Autodesk Fusion 360 part; units mm, degrees
(part 3 of 4)
  point P30 (48.244, 24.05)
  point P31 (62.214, 24.05)
  point P32 (118.094, 24.05)
  point P33 (76.184, 24.05)
  point P34 (90.154, 24.05)
  point P35 (104.124, 24.05)
  point P36 (54.673, 10.08)
  point P37 (12.673, 10.08)
  point P38 (26.673, 10.08)
  point P39 (40.673, 10.08)
  point P40 (68.673, 10.08)
  point P41 (82.673, 10.08)
  point P42 (96.673, 10.08)
  point P43 (110.673, 10.08)
  point P44 (124.673, 10.08)
  point P45 (138.673, 10.08)
  point P46 (132.064, 24.05)
  point P47 (146.034, 24.05)
  point P48 (19.024, 24.05)
  point P49 (34.274, 24.05)
  point P50 (48.244, 24.05)
  point P51 (62.214, 24.05)
  point P52 (76.184, 24.05)
  point P53 (90.154, 24.05)
  point P54 (104.124, 24.05)
  point P55 (118.094, 24.05)
  point P56 (146.034, 24.05)
  point P57 (138.673, 10.08)
  point P58 (124.673, 10.08)
  point P59 (110.673, 10.08)
  point P60 (96.673, 10.08)
  point P61 (82.673, 10.08)
  point P62 (68.673, 10.08)
  point P63 (54.673, 10.08)
  point P64 (40.673, 10.08)
  point P65 (26.673, 10.08)
  point P66 (12.673, 10.08)
  point P67 (132.064, 24.05)
  dimension "d105" = 2.7
  dimension "d106" = 2
  dimension "d371" = 1.05
  dimension "d372" = 2.7
  dimension "d373" = 2
  dimension "d374" = 1.05
  dimension "d375" = 2.7
  dimension "d376" = 2
  dimension "d377" = 1.05
  dimension "d378" = 2.7
  dimension "d379" = 2
  dimension "d380" = 1.05
  dimension "d381" = 2.7
  dimension "d382" = 2
  dimension "d383" = 1.05
  dimension "d384" = 2.7
  dimension "d385" = 2
  dimension "d386" = 1.05
  dimension "d387" = 2.7
  dimension "d388" = 2
  dimension "d389" = 1.05
  dimension "d390" = 2.7
  dimension "d391" = 2
  dimension "d392" = 1.05
  dimension "d393" = 2.7
  dimension "d394" = 2
  dimension "d395" = 1.05
  dimension "d396" = 2.7
  dimension "d397" = 2
  dimension "d398" = 1.05
  dimension "d504" = 2.7
  dimension "d505" = 2
  dimension "d506" = 1.05
  dimension "d507" = 2.7
  dimension "d508" = 2
  dimension "d509" = 1.05
  dimension "d510" = 2.7
  dimension "d511" = 2
  dimension "d512" = 1.05
  dimension "d513" = 2.7
  dimension "d514" = 2
  dimension "d515" = 1.05
  dimension "d516" = 2.7
  dimension "d517" = 2
  dimension "d518" = 1.05
  dimension "d519" = 2.7
  dimension "d520" = 2
  dimension "d521" = 1.05
  dimension "d522" = 2.7
  dimension "d523" = 2
  dimension "d524" = 1.05
  dimension "d525" = 2.7
  dimension "d526" = 2
  dimension "d527" = 1.05
  dimension "d528" = 2.7
  dimension "d529" = 2
  dimension "d530" = 1.05
  dimension "d531" = 2.7
  dimension "d532" = 2
  dimension "d533" = 1.05
  dimension "d568" = 2.7
  dimension "d569" = 2
  dimension "d570" = 1.05
  dimension "d571" = 2.7
  dimension "d572" = 2
  dimension "d573" = 1.05
  dimension "d574" = 2.7
  dimension "d575" = 2
  dimension "d576" = 1.05
  dimension "d577" = 2.7
  dimension "d578" = 2
  dimension "d579" = 1.05
  dimension "d580" = 2.7
  dimension "d581" = 2
  dimension "d582" = 1.05
  dimension "d583" = 2.7
  dimension "d584" = 2
  dimension "d585" = 1.05
  dimension "d586" = 2.7
  dimension "d587" = 2
  dimension "d588" = 1.05
  dimension "d589" = 2.7
  dimension "d590" = 2
  dimension "d591" = 1.05
  dimension "d592" = 2.7
  dimension "d593" = 2
  dimension "d594" = 1.05
  dimension "d595" = 2.7
  dimension "d596" = 2
  dimension "d597" = 1.05
  dimension "d598" = 2.7
  dimension "d599" = 2
  dimension "d600" = 1.05
  dimension "d601" = 2.7
  dimension "d602" = 2
  dimension "d603" = 1.05
  dimension "d604" = 2.7
  dimension "d605" = 2
  dimension "d606" = 1.05
  dimension "d607" = 2.7
  dimension "d608" = 2
  dimension "d609" = 1.05
  dimension "d610" = 2.7
  dimension "d611" = 2
  dimension "d612" = 1.05
  dimension "d613" = 2.7
  dimension "d614" = 2
  dimension "d615" = 1.05
  dimension "d616" = 2.7
  dimension "d617" = 2
  dimension "d618" = 1.05
  dimension "d619" = 2.7
  dimension "d620" = 2
  dimension "d621" = 1.05
  dimension "d622" = 2.7
  dimension "d623" = 2
  dimension "d624" = 1.05
  dimension "d625" = 2.7
  dimension "d626" = 2
  dimension "d627" = 1.05
  constraint midpoint L0 L4.start
  constraint midpoint L2 L4.end
  constraint midpoint L1 L5.start
  constraint midpoint L3 L5.end
  constraint vertical L6
  constraint perpendicular L5 L7
  constraint perpendicular L4 L8
  constraint perpendicular L4 L9
  constraint perpendicular L4 L11
  constraint perpendicular L7 L14
  constraint perpendicular L5 L17
  constraint equal L6 L8
  constraint equal L8 L9
  constraint equal L7 L8
  constraint symmetric L4 L8.start L8.end
  constraint symmetric L4 L10.end L11.end
  constraint symmetric L4 L9.start L9.end
  constraint symmetric L4 L13.end L14.end
  constraint symmetric L5 L6.start L6.end
  constraint symmetric L5 L16.end L17.end
  constraint symmetric L5 L7.start L7.end
  constraint collinear L0 L8
  constraint equal L11 L17
  constraint collinear L3 L6
  constraint collinear L2 L9
  constraint collinear L1 L7
  constraint equal L14 L17
  constraint parallel L7 L20
  constraint equal L17 L20
  constraint symmetric L5 L19.end L20.end
  constraint coincident L6 L22.end
  constraint coincident L3 L22.end
  constraint perpendicular L6 L22
  constraint coincident L8 L23.end
  constraint coincident L0 L23.end
  constraint coincident L9 L24.end
  constraint coincident L2 L24.end
  constraint perpendicular L9 L24
  constraint perpendicular L8 L23
  constraint coincident L7 L25.end
  constraint coincident L1 L25.end
  constraint perpendicular L7 L25
  constraint equal L23 L25
  constraint equal L22 L23
  constraint equal L23 L24
  constraint tangent L7 A0
  constraint tangent L6 A0
  constraint tangent L8 A0
  constraint vertical L27
  constraint perpendicular L38 L39
  constraint perpendicular L43 L46
  constraint perpendicular L28 L46
  constraint perpendicular L46 L47
  constraint perpendicular L34 L39
  constraint perpendicular L26 L38
  constraint equal L27 L43
  constraint equal L28 L43
  constraint equal L39 L43
  constraint symmetric L37.start L36.end L46
  constraint symmetric L37.end L32.start L46
  constraint symmetric L28.start L28.end L46
  constraint symmetric L34.start L34.end L46
  constraint symmetric L27.start L27.end L38
  constraint symmetric L26.end L26.start L38
  constraint symmetric L35.start L30.end L38
  constraint equal L26 L47
  constraint equal L26 L34
  constraint parallel L33 L39
  constraint equal L26 L33
  constraint symmetric L33.start L30.start L38
  constraint coincident L29.end L27
  constraint perpendicular L27 L29
  constraint coincident L32.end L43
  constraint coincident L41.end L28
  constraint perpendicular L28 L41
  constraint perpendicular L32 L43
  constraint coincident L42.end L39
  constraint perpendicular L39 L42
  constraint equal L32 L42
  constraint equal L29 L32
  constraint equal L32 L41
  constraint tangent L39 A1
  constraint tangent L27 A1
  constraint tangent L43 A1
  constraint coincident L38.end A1
  constraint coincident L38.start A1
  constraint coincident L46.end A1
  constraint coincident L46.start A1
  constraint tangent L28 A1
  constraint coincident P0 L46
  constraint coincident P0 L38
  constraint equal A0 A1
  constraint vertical L50
  constraint perpendicular L65 L67
  constraint perpendicular L52 L53
  constraint perpendicular L53 L61
  constraint perpendicular L53 L56
  constraint perpendicular L59 L67
  constraint perpendicular L54 L65
  constraint equal L50 L52
  constraint equal L52 L61
  constraint equal L52 L67
  constraint symmetric L51.start L48.end L53
  constraint symmetric L48.start L51.end L53
  constraint symmetric L55.end L60.start L53
  constraint symmetric L59.start L49.start L53
  constraint symmetric L50.end L50.start L65
  constraint symmetric L54.start L54.end L65
  constraint symmetric L67.start L66.end L65
  constraint equal L54 L56
  constraint equal L54 L59
  constraint parallel L67 L68
  constraint equal L54 L68
  constraint symmetric L68.start L64.start L65
  constraint coincident L62.end L50
  constraint perpendicular L50 L62
  constraint coincident L63.end L52
  constraint coincident L49.end L61
  constraint perpendicular L49 L61
  constraint perpendicular L52 L63
  constraint coincident L64.end L67
  constraint perpendicular L64 L67
  constraint equal L63 L64
  constraint equal L62 L63
  constraint equal L49 L63
  constraint tangent L67 A2
  constraint tangent L50 A2
  constraint tangent L52 A2
  constraint coincident L65.end A2
  constraint coincident L65.start A2
  constraint coincident L53.end A2
  constraint coincident L53.start A2
  constraint tangent L61 A2
  constraint coincident P1 L53
  constraint coincident P1 L65
  constraint vertical L72
  constraint perpendicular L87 L89
  constraint perpendicular L74 L75
  constraint perpendicular L75 L83
  constraint perpendicular L75 L78
  constraint perpendicular L81 L89
  constraint perpendicular L76 L87
  constraint equal L72 L74
  constraint equal L74 L83
  constraint equal L74 L89
  constraint symmetric L73.start L70.end L75
  constraint symmetric L70.start L73.end L75
  constraint symmetric L77.end L82.start L75
  constraint symmetric L81.start L71.start L75
  constraint symmetric L72.end L72.start L87
  constraint symmetric L76.start L76.end L87
  constraint symmetric L89.start L88.end L87
  constraint equal L76 L78
  constraint equal L76 L81
  constraint parallel L89 L90
  constraint equal L76 L90
  constraint symmetric L90.start L86.start L87
  constraint coincident L84.end L72
  constraint perpendicular L72 L84
  constraint coincident L85.end L74
  constraint coincident L71.end L83
  constraint perpendicular L71 L83
  constraint perpendicular L74 L85
  constraint coincident L86.end L89
  constraint perpendicular L86 L89
  constraint equal L85 L86
  constraint equal L84 L85
  constraint equal L71 L85
  constraint tangent L89 A3
  constraint tangent L72 A3
  constraint tangent L74 A3
  constraint coincident L87.end A3
  constraint coincident L87.start A3
  constraint coincident L75.end A3
  constraint coincident L75.start A3
  constraint tangent L83 A3
  constraint coincident P2 L75
  constraint coincident P2 L87
  constraint vertical L94
  constraint perpendicular L109 L111
  constraint perpendicular L96 L97
  constraint perpendicular L97 L105
  constraint perpendicular L97 L100
  constraint perpendicular L103 L111
  constraint perpendicular L98 L109
  constraint equal L94 L96
  constraint equal L96 L105
  constraint equal L96 L111
  constraint symmetric L95.start L92.end L97
  constraint symmetric L92.start L95.end L97
  constraint symmetric L99.end L104.start L97
  constraint symmetric L103.start L93.start L97
  constraint symmetric L94.end L94.start L109
  constraint symmetric L98.start L98.end L109
  constraint symmetric L111.start L110.end L109
  constraint equal L98 L100
  constraint equal L98 L103
  constraint parallel L111 L112
  constraint equal L98 L112
  constraint symmetric L112.start L108.start L109
  constraint coincident L106.end L94
  constraint perpendicular L94 L106
  constraint coincident L107.end L96
  constraint coincident L93.end L105
  constraint perpendicular L93 L105
  constraint perpendicular L96 L107
  constraint coincident L108.end L111
  constraint perpendicular L108 L111
  constraint equal L107 L108
  constraint equal L106 L107
  constraint equal L93 L107
  constraint tangent L111 A4
  constraint tangent L94 A4
  constraint tangent L96 A4
  constraint coincident L109.end A4
  constraint coincident L109.start A4
  constraint coincident L97.end A4
  constraint coincident L97.start A4
  constraint tangent L105 A4
  constraint coincident P3 L97
  constraint coincident P3 L109
  constraint vertical L116
  constraint perpendicular L131 L133
  constraint perpendicular L118 L119
  constraint perpendicular L119 L127
  constraint perpendicular L119 L122
  constraint perpendicular L125 L133
  constraint perpendicular L120 L131
  constraint equal L116 L118
  constraint equal L118 L127
  constraint equal L118 L133
  constraint symmetric L117.start L114.end L119
  constraint symmetric L114.start L117.end L119
  constraint symmetric L121.end L126.start L119
  constraint symmetric L125.start L115.start L119
  constraint symmetric L116.end L116.start L131
  constraint symmetric L120.start L120.end L131
  constraint symmetric L133.start L132.end L131
  constraint equal L120 L122
  constraint equal L120 L125
  constraint parallel L133 L134
  constraint equal L120 L134
  constraint symmetric L134.start L130.start L131
  constraint coincident L128.end L116
  constraint perpendicular L116 L128
  constraint coincident L129.end L118
  constraint coincident L115.end L127
  constraint perpendicular L115 L127
  constraint perpendicular L118 L129
  constraint coincident L130.end L133
  constraint perpendicular L130 L133
  constraint equal L129 L130
  constraint equal L128 L129
  constraint equal L115 L129
  constraint tangent L133 A5
  constraint tangent L116 A5
  constraint tangent L118 A5
  constraint coincident L131.end A5
  constraint coincident L131.start A5
  constraint coincident L119.end A5
  constraint coincident L119.start A5
  constraint tangent L127 A5
  constraint coincident P4 L119
  constraint coincident P4 L131
  constraint vertical L138
  constraint perpendicular L153 L155
  constraint perpendicular L140 L141
  constraint perpendicular L141 L149
  constraint perpendicular L141 L144
  constraint perpendicular L147 L155
  constraint perpendicular L142 L153
  constraint equal L138 L140
  constraint equal L140 L149
  constraint equal L140 L155
  constraint symmetric L139.start L136.end L141
  constraint symmetric L136.start L139.end L141
  constraint symmetric L143.end L148.start L141
  constraint symmetric L147.start L137.start L141
  constraint symmetric L138.end L138.start L153
  constraint symmetric L142.start L142.end L153
  constraint symmetric L155.start L154.end L153
  constraint equal L142 L144
  constraint equal L142 L147
  constraint parallel L155 L156
  constraint equal L142 L156
  constraint symmetric L156.start L152.start L153
  constraint coincident L150.end L138
  constraint perpendicular L138 L150
  constraint coincident L151.end L140
  constraint coincident L137.end L149
  constraint perpendicular L137 L149
  constraint perpendicular L140 L151
  constraint coincident L152.end L155
  constraint perpendicular L152 L155
  constraint equal L151 L152
  constraint equal L150 L151
  constraint equal L137 L151
  constraint tangent L155 A6
  constraint tangent L138 A6
  constraint tangent L140 A6
  constraint coincident L153.end A6
  constraint coincident L153.start A6
  constraint coincident L141.end A6
  constraint coincident L141.start A6
  constraint tangent L149 A6
  constraint coincident P5 L141
  constraint coincident P5 L153
  constraint vertical L160
  constraint perpendicular L175 L177
  constraint perpendicular L162 L163
  constraint perpendicular L163 L171
  constraint perpendicular L163 L166
  constraint perpendicular L169 L177
  constraint perpendicular L164 L175
  constraint equal L160 L162
  constraint equal L162 L171
  constraint equal L162 L177
  constraint symmetric L161.start L158.end L163
  constraint symmetric L158.start L161.end L163
  constraint symmetric L165.end L170.start L163
  constraint symmetric L169.start L159.start L163
  constraint symmetric L160.end L160.start L175
  constraint symmetric L164.start L164.end L175
  constraint symmetric L177.start L176.end L175
  constraint equal L164 L166
  constraint equal L164 L169
  constraint parallel L177 L178
  constraint equal L164 L178
  constraint symmetric L178.start L174.start L175
  constraint coincident L172.end L160
  constraint perpendicular L160 L172
  constraint coincident L173.end L162
  constraint coincident L159.end L171
  constraint perpendicular L159 L171
  constraint perpendicular L162 L173
  constraint coincident L174.end L177
  constraint perpendicular L174 L177
  constraint equal L173 L174
  constraint equal L172 L173
  constraint equal L159 L173
  constraint tangent L177 A7
  constraint tangent L160 A7
  constraint tangent L162 A7
  constraint coincident L175.end A7
  constraint coincident L175.start A7
  constraint coincident L163.end A7
  constraint coincident L163.start A7
  constraint tangent L171 A7
  constraint coincident P6 L163
  constraint coincident P6 L175
  constraint vertical L182
  constraint perpendicular L197 L199
  constraint perpendicular L184 L185
  constraint perpendicular L185 L193
  constraint perpendicular L185 L188
  constraint perpendicular L191 L199
  constraint perpendicular L186 L197
  constraint equal L182 L184
  constraint equal L184 L193
  constraint equal L184 L199
  constraint symmetric L183.start L180.end L185
  constraint symmetric L180.start L183.end L185
  constraint symmetric L187.end L192.start L185
  constraint symmetric L191.start L181.start L185
  constraint symmetric L182.end L182.start L197
  constraint symmetric L186.start L186.end L197
  constraint symmetric L199.start L198.end L197
  constraint equal L186 L188
  constraint equal L186 L191
  constraint parallel L199 L200
  constraint equal L186 L200
  constraint symmetric L200.start L196.start L197
  constraint coincident L194.end L182
  constraint perpendicular L182 L194
  constraint coincident L195.end L184
  constraint coincident L181.end L193
  constraint perpendicular L181 L193
  constraint perpendicular L184 L195
  constraint coincident L196.end L199
  constraint perpendicular L196 L199
  constraint equal L195 L196
  constraint equal L194 L195
  constraint equal L181 L195
  constraint tangent L199 A8
  constraint tangent L182 A8
  constraint tangent L184 A8
  constraint coincident L197.end A8
  constraint coincident L197.start A8
  constraint coincident L185.end A8
  constraint coincident L185.start A8
  constraint tangent L193 A8
  constraint coincident P7 L185
  constraint coincident P7 L197
  constraint vertical L204
  constraint perpendicular L219 L221
  constraint perpendicular L206 L207
  constraint perpendicular L207 L215
  constraint perpendicular L207 L210
  constraint perpendicular L213 L221
  constraint perpendicular L208 L219
  constraint equal L204 L206
  constraint equal L206 L215
  constraint equal L206 L221
  constraint symmetric L205.start L202.end L207
  constraint symmetric L202.start L205.end L207
  constraint symmetric L209.end L214.start L207
  constraint symmetric L213.start L203.start L207
  constraint symmetric L204.end L204.start L219
  constraint symmetric L208.start L208.end L219
  constraint symmetric L221.start L220.end L219
  constraint equal L208 L210
  constraint equal L208 L213
  constraint parallel L221 L222
  constraint equal L208 L222
  constraint symmetric L222.start L218.start L219
  constraint coincident L216.end L204
  constraint perpendicular L204 L216
  constraint coincident L217.end L206
  constraint coincident L203.end L215
  constraint perpendicular L203 L215
  constraint perpendicular L206 L217
  constraint coincident L218.end L221
  constraint perpendicular L218 L221
  constraint equal L217 L218
  constraint equal L216 L217
  constraint equal L203 L217
  constraint tangent L221 A9
  constraint tangent L204 A9
  constraint tangent L206 A9
  constraint coincident L219.end A9
  constraint coincident L219.start A9
  constraint coincident L207.end A9
  constraint coincident L207.start A9
  constraint tangent L215 A9
  constraint coincident P8 L207
  constraint coincident P8 L219
  constraint coincident P0 A1.centre
  constraint coincident P1 A2.centre
  constraint equal A0 A2
  constraint coincident P2 A3.centre
  constraint equal A0 A3
  constraint coincident P3 A4.centre
  constraint coincident P4 A5.centre
  constraint coincident P5 A6.centre
  constraint coincident P6 A7.centre
  constraint coincident P7 A8.centre
  constraint coincident P8 A9.centre
  constraint equal A0 A4
  constraint equal A0 A9
  constraint equal A0 A8
  constraint equal A0 A7
  constraint equal A0 A6
  constraint equal A0 A5
  constraint vertical L227
  constraint perpendicular L234 L236
  constraint perpendicular L235 L238
  constraint perpendicular L238 L241
  constraint perpendicular L238 L243
  constraint perpendicular L228 L234
  constraint perpendicular L229 L236
  constraint equal L227 L235
  constraint equal L235 L241
  constraint equal L234 L235
  constraint symmetric L224.start L235.end L238
  constraint symmetric L230.start L224.end L238
  constraint symmetric L232.start L237.end L238
  constraint symmetric L228.start L228.end L238
  constraint symmetric L227.end L227.start L236
  constraint symmetric L229.start L229.end L236
  constraint symmetric L234.start L234.end L236
  constraint equal L229 L243
  constraint equal L228 L229
  constraint parallel L226 L234
  constraint equal L226 L229
  constraint symmetric L226.start L225.start L236
  constraint coincident L245.end L227
  constraint perpendicular L227 L245
  constraint coincident L230.end L235
  constraint coincident L233.end L241
  constraint perpendicular L233 L241
  constraint perpendicular L230 L235
  constraint coincident L225.end L234
  constraint perpendicular L225 L234
  constraint equal L225 L230
  constraint equal L230 L245
  constraint equal L230 L233
  constraint tangent A10 L234
  constraint tangent A10 L227
  constraint tangent A10 L235
  constraint coincident L236.end A10
  constraint coincident L236.start A10
  constraint coincident L238.end A10
  constraint coincident L238.start A10
  constraint tangent A10 L241
  constraint coincident P19 L238
  constraint coincident P19 L236
  constraint coincident P19 P9
  constraint vertical L249
  constraint perpendicular L256 L258
  constraint perpendicular L257 L260
  constraint perpendicular L260 L263
  constraint perpendicular L260 L265
  constraint perpendicular L250 L256
  constraint perpendicular L251 L258
  constraint equal L249 L257
  constraint equal L257 L263
  constraint equal L256 L257
  constraint symmetric L246.start L257.end L260
  constraint symmetric L252.start L246.end L260
  constraint symmetric L254.start L259.end L260
  constraint symmetric L250.start L250.end L260
  constraint symmetric L249.end L249.start L258
  constraint symmetric L251.start L251.end L258
  constraint symmetric L256.start L256.end L258
  constraint equal L251 L265
  constraint equal L250 L251
  constraint parallel L248 L256
  constraint equal L248 L251
  constraint symmetric L248.start L247.start L258
  constraint coincident L267.end L249
  constraint perpendicular L249 L267
  constraint coincident L252.end L257
  constraint coincident L255.end L263
  constraint perpendicular L255 L263
  constraint perpendicular L252 L257
  constraint coincident L247.end L256
  constraint perpendicular L247 L256
  constraint equal L247 L252
  constraint equal L252 L267
  constraint equal L252 L255
  constraint tangent A11 L256
  constraint tangent A11 L249
  constraint tangent A11 L257
  constraint coincident L258.end A11
  constraint coincident L258.start A11
  constraint coincident L260.end A11
  constraint coincident L260.start A11
  constraint tangent A11 L263
  constraint coincident P27 L260
  constraint coincident P27 L258
  constraint coincident P27 P10
  constraint vertical L271
  constraint perpendicular L278 L280
  constraint perpendicular L279 L282
  constraint perpendicular L282 L285
  constraint perpendicular L282 L287
  constraint perpendicular L272 L278
  constraint perpendicular L273 L280
  constraint equal L271 L279
  constraint equal L279 L285
  constraint equal L278 L279
  constraint symmetric L268.start L279.end L282
  constraint symmetric L274.start L268.end L282
  constraint symmetric L276.start L281.end L282
  constraint symmetric L272.start L272.end L282
  constraint symmetric L271.end L271.start L280
  constraint symmetric L273.start L273.end L280
  constraint symmetric L278.start L278.end L280
  constraint equal L273 L287
  constraint equal L272 L273
  constraint parallel L270 L278
  constraint equal L270 L273
  constraint symmetric L270.start L269.start L280
  constraint coincident L289.end L271
  constraint perpendicular L271 L289
  constraint coincident L274.end L279
  constraint coincident L277.end L285
  constraint perpendicular L277 L285
  constraint perpendicular L274 L279
  constraint coincident L269.end L278
  constraint perpendicular L269 L278
  constraint equal L269 L274
  constraint equal L274 L289
  constraint equal L274 L277
  constraint tangent A12 L278
  constraint tangent A12 L271
  constraint tangent A12 L279
  constraint coincident L280.end A12
  constraint coincident L280.start A12
  constraint coincident L282.end A12
  constraint coincident L282.start A12
  constraint tangent A12 L285
  constraint coincident P26 L282
  constraint coincident P26 L280
  constraint coincident P26 P11
  constraint vertical L293
  constraint perpendicular L300 L302
  constraint perpendicular L301 L304
  constraint perpendicular L304 L307
  constraint perpendicular L304 L309
  constraint perpendicular L294 L300
  constraint perpendicular L295 L302
  constraint equal L293 L301
  constraint equal L301 L307
  constraint equal L300 L301
  constraint symmetric L290.start L301.end L304
  constraint symmetric L296.start L290.end L304
  constraint symmetric L298.start L303.end L304
  constraint symmetric L294.start L294.end L304
  constraint symmetric L293.end L293.start L302
  constraint symmetric L295.start L295.end L302
  constraint symmetric L300.start L300.end L302
  constraint equal L295 L309
  constraint equal L294 L295
  constraint parallel L292 L300
  constraint equal L292 L295
  constraint symmetric L292.start L291.start L302
  constraint coincident L311.end L293
  constraint perpendicular L293 L311
  constraint coincident L296.end L301
  constraint coincident L299.end L307
  constraint perpendicular L299 L307
  constraint perpendicular L296 L301
  constraint coincident L291.end L300
  constraint perpendicular L291 L300
  constraint equal L291 L296
  constraint equal L296 L311
  constraint equal L296 L299
  constraint tangent A13 L300
  constraint tangent A13 L293
  constraint tangent A13 L301
  constraint coincident L302.end A13
  constraint coincident L302.start A13
  constraint coincident L304.end A13
  constraint coincident L304.start A13
  constraint tangent A13 L307
  constraint coincident P25 L304
  constraint coincident P25 L302
  constraint coincident P25 P12
  constraint vertical L315
  constraint perpendicular L322 L324
  constraint perpendicular L323 L326
  constraint perpendicular L326 L329
  constraint perpendicular L326 L331
  constraint perpendicular L316 L322
  constraint perpendicular L317 L324
  constraint equal L315 L323
  constraint equal L323 L329
  constraint equal L322 L323
  constraint symmetric L312.start L323.end L326
  constraint symmetric L318.start L312.end L326
  constraint symmetric L320.start L325.end L326
  constraint symmetric L316.start L316.end L326
  constraint symmetric L315.end L315.start L324
  constraint symmetric L317.start L317.end L324
  constraint symmetric L322.start L322.end L324
  constraint equal L317 L331
  constraint equal L316 L317
  constraint parallel L314 L322
  constraint equal L314 L317
  constraint symmetric L314.start L313.start L324
  constraint coincident L333.end L315
  constraint perpendicular L315 L333
  constraint coincident L318.end L323
  constraint coincident L321.end L329
  constraint perpendicular L321 L329
  constraint perpendicular L318 L323
  constraint coincident L313.end L322
  constraint perpendicular L313 L322
  constraint equal L313 L318
  constraint equal L318 L333
  constraint equal L318 L321
  constraint tangent A14 L322
  constraint tangent A14 L315
  constraint tangent A14 L323
  constraint coincident L324.end A14
  constraint coincident L324.start A14
  constraint coincident L326.end A14
  constraint coincident L326.start A14
  constraint tangent A14 L329
  constraint coincident P18 L326
  constraint coincident P18 L324
  constraint vertical L337
  constraint perpendicular L344 L346
  constraint perpendicular L345 L348
  constraint perpendicular L348 L351
  constraint perpendicular L348 L353
  constraint perpendicular L338 L344
  constraint perpendicular L339 L346
  constraint equal L337 L345
  constraint equal L345 L351
  constraint equal L344 L345
  constraint symmetric L334.start L345.end L348
  constraint symmetric L340.start L334.end L348
  constraint symmetric L342.start L347.end L348
  constraint symmetric L338.start L338.end L348
  constraint symmetric L337.end L337.start L346
  constraint symmetric L339.start L339.end L346
  constraint symmetric L344.start L344.end L346
  constraint equal L339 L353
  constraint equal L338 L339
  constraint parallel L336 L344
  constraint equal L336 L339
  constraint symmetric L336.start L335.start L346
  constraint coincident L355.end L337
  constraint perpendicular L337 L355
  constraint coincident L340.end L345
  constraint coincident L343.end L351
  constraint perpendicular L343 L351
  constraint perpendicular L340 L345
  constraint coincident L335.end L344
  constraint perpendicular L335 L344
  constraint equal L335 L340
  constraint equal L340 L355
  constraint equal L340 L343
  constraint tangent A15 L344
  constraint tangent A15 L337
  constraint tangent A15 L345
  constraint coincident L346.end A15
  constraint coincident L346.start A15
  constraint coincident L348.end A15
  constraint coincident L348.start A15
  constraint tangent A15 L351
  constraint coincident P24 L348
  constraint coincident P24 L346
  constraint coincident P24 P13
  constraint vertical L359
  constraint perpendicular L366 L368
  constraint perpendicular L367 L370
  constraint perpendicular L370 L373
  constraint perpendicular L370 L375
  constraint perpendicular L360 L366
  constraint perpendicular L361 L368
  constraint equal L359 L367
  constraint equal L367 L373
  constraint equal L366 L367
  constraint symmetric L356.start L367.end L370
  constraint symmetric L362.start L356.end L370
  constraint symmetric L364.start L369.end L370
  constraint symmetric L360.start L360.end L370
  constraint symmetric L359.end L359.start L368
  constraint symmetric L361.start L361.end L368
  constraint symmetric L366.start L366.end L368
  constraint equal L361 L375
  constraint equal L360 L361
  constraint parallel L358 L366
  constraint equal L358 L361
  constraint symmetric L358.start L357.start L368
  constraint coincident L377.end L359
  constraint perpendicular L359 L377
  constraint coincident L362.end L367
  constraint coincident L365.end L373
  constraint perpendicular L365 L373
  constraint perpendicular L362 L367
  constraint coincident L357.end L366
  constraint perpendicular L357 L366
  constraint equal L357 L362
  constraint equal L362 L377
  constraint equal L362 L365
  constraint tangent A16 L366
  constraint tangent A16 L359
  constraint tangent A16 L367
  constraint coincident L368.end A16
  constraint coincident L368.start A16
  constraint coincident L370.end A16
  constraint coincident L370.start A16
  constraint tangent A16 L373
  constraint coincident P23 L370
  constraint coincident P23 L368
  constraint coincident P23 P14
  constraint vertical L381
  constraint perpendicular L388 L390
  constraint perpendicular L389 L392
  constraint perpendicular L392 L395
  constraint perpendicular L392 L397
  constraint perpendicular L382 L388
  constraint perpendicular L383 L390
  constraint equal L381 L389
  constraint equal L389 L395
  constraint equal L388 L389
  constraint symmetric L378.start L389.end L392
  constraint symmetric L384.start L378.end L392
  constraint symmetric L386.start L391.end L392
  constraint symmetric L382.start L382.end L392
  constraint symmetric L381.end L381.start L390
  constraint symmetric L383.start L383.end L390
  constraint symmetric L388.start L388.end L390
  constraint equal L383 L397
  constraint equal L382 L383
  constraint parallel L380 L388
  constraint equal L380 L383
  constraint symmetric L380.start L379.start L390
  constraint coincident L399.end L381
  constraint perpendicular L381 L399
  constraint coincident L384.end L389
  constraint coincident L387.end L395
  constraint perpendicular L387 L395
  constraint perpendicular L384 L389
  constraint coincident L379.end L388
  constraint perpendicular L379 L388
  constraint equal L379 L384
  constraint equal L384 L399
  constraint equal L384 L387
  constraint tangent A17 L388
  constraint tangent A17 L381
  constraint tangent A17 L389
  constraint coincident L390.end A17
  constraint coincident L390.start A17
  constraint coincident L392.end A17
  constraint coincident L392.start A17
  constraint tangent A17 L395
  constraint coincident P22 L392
  constraint coincident P22 L390
  constraint coincident P22 P15
  constraint vertical L403
  constraint perpendicular L410 L412
  constraint perpendicular L411 L414
  constraint perpendicular L414 L417
  constraint perpendicular L414 L419
  constraint perpendicular L404 L410
  constraint perpendicular L405 L412
  constraint equal L403 L411
  constraint equal L411 L417
  constraint equal L410 L411
  constraint symmetric L400.start L411.end L414
  constraint symmetric L406.start L400.end L414
  constraint symmetric L408.start L413.end L414
  constraint symmetric L404.start L404.end L414
  constraint symmetric L403.end L403.start L412
  constraint symmetric L405.start L405.end L412
  constraint symmetric L410.start L410.end L412
  constraint equal L405 L419
  constraint equal L404 L405
  constraint parallel L402 L410
  constraint equal L402 L405
  constraint symmetric L402.start L401.start L412
  constraint coincident L421.end L403
  constraint perpendicular L403 L421
  constraint coincident L406.end L411
  constraint coincident L409.end L417
  constraint perpendicular L409 L417
  constraint perpendicular L406 L411
  constraint coincident L401.end L410
  constraint perpendicular L401 L410
  constraint equal L401 L406
  constraint equal L406 L421
  constraint equal L406 L409
  constraint tangent A18 L410
  constraint tangent A18 L403
  constraint tangent A18 L411
  constraint coincident L412.end A18
  constraint coincident L412.start A18
  constraint coincident L414.end A18
  constraint coincident L414.start A18
  constraint tangent A18 L417
  constraint coincident P21 L414
  constraint coincident P21 L412
  constraint coincident P21 P16
  constraint vertical L425
  constraint perpendicular L432 L434
  constraint perpendicular L433 L436
  constraint perpendicular L436 L439
  constraint perpendicular L436 L441
  constraint perpendicular L426 L432
  constraint perpendicular L427 L434
  constraint equal L425 L433
  constraint equal L433 L439
  constraint equal L432 L433
  constraint symmetric L422.start L433.end L436
  constraint symmetric L428.start L422.end L436
  constraint symmetric L430.start L435.end L436
  constraint symmetric L426.start L426.end L436
  constraint symmetric L425.end L425.start L434
  constraint symmetric L427.start L427.end L434
  constraint symmetric L432.start L432.end L434
  constraint equal L427 L441
  constraint equal L426 L427
  constraint parallel L424 L432
  constraint equal L424 L427
  constraint symmetric L424.start L423.start L434
  constraint coincident L443.end L425
  constraint perpendicular L425 L443
  constraint coincident L428.end L433
  constraint coincident L431.end L439
  constraint perpendicular L431 L439
  constraint perpendicular L428 L433
  constraint coincident L423.end L432
  constraint perpendicular L423 L432
  constraint equal L423 L428
  constraint equal L428 L443
  constraint equal L428 L431
  constraint tangent A19 L432
  constraint tangent A19 L425
  constraint tangent A19 L433
  constraint coincident L434.end A19
  constraint coincident L434.start A19
  constraint coincident L436.end A19
  constraint coincident L436.start A19
  constraint tangent A19 L439
  constraint coincident P20 L436
  constraint coincident P20 L434
  constraint coincident P20 P17
  constraint coincident P18 A14.centre
  constraint equal A14 A20
  constraint equal A10 A21
  constraint equal A11 A22
  constraint equal A12 A23
  constraint equal A13 A24
  constraint equal A15 A25
  constraint equal A16 A26
  constraint equal A17 A27
  constraint equal A18 A28
  constraint equal A19 A29
  constraint vertical L464
  constraint perpendicular L446 L448
  constraint perpendicular L452 L463
  constraint perpendicular L453 L463
  constraint perpendicular L462 L463
  constraint perpendicular L448 L456
  constraint perpendicular L446 L465
  constraint equal L452 L464
  constraint equal L452 L453
  constraint equal L448 L452
  constraint symmetric L450.end L452.start L463
  constraint symmetric L450.start L459.end L463
  constraint symmetric L447.start L444.end L463
  constraint symmetric L444.start L447.end L463
  constraint symmetric L460.end L461.start L446
  constraint symmetric L461.end L458.start L446
  constraint symmetric L448.start L448.end L446
  constraint equal L462 L465
  constraint equal L456 L465
  constraint parallel L448 L451
  constraint equal L451 L465
  constraint symmetric L451.end L449.end L446
  constraint coincident L458.end L464
  constraint perpendicular L458 L464
  constraint coincident L457.end L452
  constraint coincident L445.end L453
  constraint perpendicular L445 L453
  constraint perpendicular L452 L457
  constraint coincident L454.end L448
  constraint perpendicular L448 L454
  constraint equal L454 L457
  constraint equal L457 L458
  constraint equal L445 L457
  constraint tangent L448 A30
  constraint tangent A30 L464
  constraint tangent L452 A30
  constraint coincident L446.end A30
  constraint coincident L446.start A30
  constraint coincident L463.end A30
  constraint coincident L463.start A30
  constraint tangent A30 L453
  constraint coincident P48 L463
  constraint coincident P48 L446
  constraint coincident P48 P28
  constraint vertical L474
  constraint perpendicular L468 L472
  constraint perpendicular L481 L485
  constraint perpendicular L470 L485
  constraint perpendicular L482 L485
  constraint perpendicular L472 L480
  constraint perpendicular L468 L475
  constraint equal L474 L481
  constraint equal L470 L481
  constraint equal L472 L481
  constraint symmetric L477.end L481.start L485
  constraint symmetric L477.start L482.start L485
  constraint symmetric L470.end L466.end L485
  constraint symmetric L466.start L476.end L485
  constraint symmetric L474.start L469.start L468
  constraint symmetric L469.end L475.end L468
  constraint symmetric L472.start L471.end L468
  constraint equal L475 L482
  constraint equal L475 L480
  constraint parallel L472 L487
  constraint equal L475 L487
  constraint symmetric L467.start L473.end L468
  constraint coincident L479.end L474
  constraint perpendicular L474 L479
  constraint coincident L478.end L481
  constraint coincident L483.end L470
  constraint perpendicular L470 L483
  constraint perpendicular L478 L481
  constraint coincident L467.end L472
  constraint perpendicular L467 L472
  constraint equal L467 L478
  constraint equal L478 L479
  constraint equal L478 L483
  constraint tangent L472 A31
  constraint tangent L474 A31
  constraint tangent A31 L481
  constraint coincident L468.end A31
  constraint coincident L468.start A31
  constraint coincident L485.end A31
  constraint coincident L485.start A31
  constraint tangent L470 A31
  constraint coincident P49 L485
  constraint coincident P49 L468
  constraint coincident P49 P29
  constraint vertical L522
  constraint perpendicular L488 L530
  constraint perpendicular L499 L526
  constraint perpendicular L492 L526
  constraint perpendicular L510 L526
  constraint perpendicular L488 L503
  constraint perpendicular L505 L530
  constraint equal L499 L522
  constraint equal L492 L499
  constraint equal L488 L499
  constraint symmetric L495.end L499.start L526
  constraint symmetric L495.start L510.start L526
  constraint symmetric L492.end L492.start L526
  constraint symmetric L503.end L497.end L526
  constraint symmetric L506.end L508.start L530
  constraint symmetric L505.start L504.start L530
  constraint symmetric L488.start L488.end L530
  constraint equal L505 L510
  constraint equal L503 L505
  constraint parallel L488 L493
  constraint equal L493 L505
  constraint symmetric L493.end L491.end L530
  constraint coincident L504.end L522
  constraint perpendicular L504 L522
  constraint coincident L528.end L499
  constraint coincident L519.end L492
  constraint perpendicular L492 L519
  constraint perpendicular L499 L528
  constraint coincident L498.end L488
  constraint perpendicular L488 L498
  constraint equal L498 L528
  constraint equal L504 L528
  constraint equal L519 L528
  constraint tangent L488 A32
  constraint tangent A32 L522
  constraint tangent L499 A32
  constraint coincident L530.end A32
  constraint coincident L530.start A32
  constraint coincident L526.end A32
  constraint coincident L526.start A32
  constraint tangent L492 A32
  constraint coincident P50 L526
  constraint coincident P50 L530
  constraint coincident P50 P30
  constraint vertical L517
  constraint perpendicular L489 L524
  constraint perpendicular L513 L520
  constraint perpendicular L501 L520
  constraint perpendicular L496 L520
  constraint perpendicular L507 L524
  constraint perpendicular L489 L502
  constraint equal L513 L517
  constraint equal L501 L513
  constraint equal L513 L524
  constraint symmetric L513.start L513.end L520
  constraint symmetric L496.start L496.end L520
  constraint symmetric L494.end L501.end L520
  constraint symmetric L494.start L507.start L520
  constraint symmetric L500.end L509.start L489
  constraint symmetric L502.start L490.start L489
  constraint symmetric L511.end L516.start L489
  constraint equal L496 L502
  constraint equal L502 L507
  constraint parallel L524 L525
  constraint equal L502 L525
  constraint symmetric L511.start L516.end L489
  constraint coincident L490.end L517
  constraint perpendicular L490 L517
  constraint coincident L523.end L513
  constraint coincident L521.end L501
  constraint perpendicular L501 L521
  constraint perpendicular L513 L523
  constraint coincident L514.end L524
  constraint perpendicular L514 L524
  constraint equal L514 L523
  constraint equal L490 L523
  constraint equal L521 L523
  constraint tangent A33 L524
  constraint tangent L517 A33
  constraint tangent L513 A33
  constraint coincident L489.end A33
  constraint coincident L489.start A33
  constraint coincident L520.end A33
  constraint coincident L520.start A33
  constraint tangent L501 A33
  constraint coincident P51 L520
  constraint coincident P51 L489
  constraint coincident P51 P31
  constraint vertical L574
  constraint perpendicular L535 L578
  constraint perpendicular L559 L581
  constraint perpendicular L554 L559
  constraint perpendicular L559 L588
  constraint perpendicular L535 L594
  constraint perpendicular L578 L598
  constraint equal L574 L581
  constraint equal L554 L581
  constraint equal L535 L581
  constraint symmetric L542.end L581.start L559
  constraint symmetric L542.start L588.start L559
  constraint symmetric L548.start L554.start L559
  constraint symmetric L582.start L548.end L559
  constraint symmetric L569.end L574.end L578
  constraint symmetric L575.end L569.start L578
  constraint symmetric L535.start L533.end L578
  constraint equal L588 L598
  constraint equal L594 L598
  constraint parallel L535 L560
  constraint equal L560 L598
  constraint symmetric L533.start L545.end L578
  constraint coincident L583.end L574
  constraint perpendicular L574 L583
  constraint coincident L561.end L581
  constraint coincident L582.end L554
  constraint perpendicular L554 L582
  constraint perpendicular L561 L581
  constraint coincident L534.end L535
  constraint perpendicular L534 L535
  constraint equal L534 L561
  constraint equal L561 L583
  constraint equal L561 L582
  constraint tangent L535 A36
  constraint tangent L574 A36
  constraint tangent L581 A36
  constraint coincident L578.end A36
  constraint coincident L578.start A36
  constraint coincident L559.end A36
  constraint coincident L559.start A36
  constraint tangent L554 A36
  constraint coincident P52 L559
  constraint coincident P52 L578
  constraint coincident P52 P33
  constraint vertical L602
  constraint perpendicular L532 L536
  constraint perpendicular L553 L576
  constraint perpendicular L553 L571
  constraint perpendicular L553 L609
  constraint perpendicular L532 L566
  constraint perpendicular L536 L567
  constraint equal L576 L602
  constraint equal L571 L576
  constraint equal L532 L576
  constraint symmetric L576.start L539.end L553
  constraint symmetric L601.end L539.start L553
  constraint symmetric L547.end L550.start L553
  constraint symmetric L547.start L550.end L553
  constraint symmetric L538.end L556.start L536
  constraint symmetric L556.end L538.start L536
  constraint symmetric L532.end L532.start L536
  constraint equal L567 L609
  constraint equal L566 L567
  constraint parallel L532 L570
  constraint equal L567 L570
  constraint symmetric L570.end L570.start L536
  constraint coincident L558.end L602
  constraint perpendicular L558 L602
  constraint coincident L540.end L576
  constraint coincident L551.end L571
  constraint perpendicular L551 L571
  constraint perpendicular L540 L576
  constraint coincident L573.end L532
  constraint perpendicular L532 L573
  constraint equal L540 L573
  constraint equal L540 L558
  constraint equal L540 L551
  constraint tangent L532 A35
  constraint tangent A35 L602
  constraint tangent A35 L576
  constraint coincident L536.end A35
  constraint coincident L536.start A35
  constraint coincident L553.end A35
  constraint coincident L553.start A35
  constraint tangent A35 L571
  constraint coincident P53 L553
  constraint coincident P53 L536
  constraint coincident P53 P34
  constraint vertical L564
  constraint perpendicular L546 L600
  constraint perpendicular L549 L580
  constraint perpendicular L580 L590
  constraint perpendicular L562 L580
  constraint perpendicular L544 L546
  constraint perpendicular L579 L600
  constraint equal L549 L564
  constraint equal L549 L590
  constraint equal L546 L549
  constraint symmetric L549.end L549.start L580
  constraint symmetric L555.start L562.start L580
  constraint symmetric L537.start L563.end L580
  constraint symmetric L544.end L537.end L580
  constraint symmetric L541.end L543.start L600
  constraint symmetric L543.end L541.start L600
  constraint symmetric L546.end L546.start L600
  constraint equal L562 L579
  constraint equal L544 L579
  constraint parallel L546 L585
  constraint equal L579 L585
  constraint symmetric L552.start L568.end L600
  constraint coincident L557.end L564
  constraint perpendicular L557 L564
  constraint coincident L555.end L549
  constraint coincident L599.end L590
  constraint perpendicular L590 L599
  constraint perpendicular L549 L555
  constraint coincident L552.end L546
  constraint perpendicular L546 L552
  constraint equal L552 L555
  constraint equal L555 L557
  constraint equal L555 L599
  constraint tangent A34 L546
  constraint tangent A34 L564
  constraint tangent A34 L549
  constraint coincident L600.end A34
  constraint coincident L600.start A34
  constraint coincident L580.end A34
  constraint coincident L580.start A34
  constraint tangent A34 L590
  constraint coincident P54 L580
  constraint coincident P54 L600
  constraint coincident P54 P35
  constraint vertical L616
  constraint perpendicular L605 L618
  constraint perpendicular L572 L611
  constraint perpendicular L572 L610
  constraint perpendicular L572 L589
  constraint perpendicular L605 L608
  constraint perpendicular L618 L619
  constraint equal L611 L616
  constraint equal L610 L611
  constraint equal L605 L611
  constraint symmetric L591.start L586.end L572
  constraint symmetric L589.start L586.start L572
  constraint symmetric L610.start L610.end L572
  constraint symmetric L608.end L608.start L572
  constraint symmetric L565.end L584.start L618
  constraint symmetric L584.end L565.start L618
  constraint symmetric L605.end L577.start L618
  constraint equal L589 L619
  constraint equal L608 L619
  constraint parallel L593 L605
  constraint equal L593 L619
  constraint symmetric L577.end L593.end L618
  constraint coincident L607.end L616
  constraint perpendicular L607 L616
  constraint coincident L615.end L611
  constraint coincident L612.end L610
  constraint perpendicular L610 L612
  constraint perpendicular L611 L615
  constraint coincident L597.end L605
  constraint perpendicular L597 L605
  constraint equal L597 L615
  constraint equal L607 L615
  constraint equal L612 L615
  constraint tangent L605 A37
  constraint tangent A37 L616
  constraint tangent L611 A37
  constraint coincident L618.end A37
  constraint coincident L618.start A37
  constraint coincident L572.end A37
  constraint coincident L572.start A37
  constraint tangent L610 A37
  constraint coincident P55 L572
  constraint coincident P55 L618
  constraint coincident P55 P32
  constraint vertical L690
  constraint perpendicular L658 L694
  constraint perpendicular L622 L768
  constraint perpendicular L622 L734
  constraint perpendicular L622 L732
  constraint perpendicular L658 L696
  constraint perpendicular L694 L709
  constraint equal L690 L768
  constraint equal L734 L768
  constraint equal L658 L768
  constraint symmetric L652.end L663.start L622
  constraint symmetric L626.start L663.end L622
  constraint symmetric L708.start L688.end L622
  constraint symmetric L688.start L696.start L622
  constraint symmetric L690.start L690.end L694
  constraint symmetric L709.start L683.start L694
  constraint symmetric L658.start L639.end L694
  constraint equal L709 L732
  constraint equal L696 L709
  constraint parallel L658 L681
  constraint equal L681 L709
  constraint symmetric L630.start L675.end L694
  constraint coincident L683.end L690
  constraint perpendicular L683 L690
  constraint coincident L626.end L768